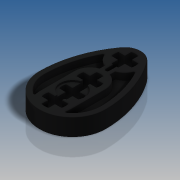
# Autodesk Inventor part: 6575-Black
Saved by Autodesk Inventor 2016 SP2 (Build 200236200, 236)
## iProperties
Created: 2015-01-12
Part Number: 6575-Black
Material: ABS Plastic
Document SubType Name: Modeling
Designer: D. Kohfeld
Density: 1.06 g/cm^3
Appearance: Black
Mass: 0.667179 g
Surface Area: 11.7051 cm^2
Volume: 0.629414 cm^3
Author: D. Kohfeld
Autodesk Inventor part; units mm, degrees
ref_plane "YZ Plane" through (0, 0, 0) normal (1, 0, 0) x (0, 1, 0)
ref_plane "XZ Plane" through (0, 0, 0) normal (0, 1, 0) x (-1, 0, 0)
ref_plane "XY Plane" through (0, 0, 0) normal (0, 0, 1) x (1, 0, 0)
sketch "Sketch2" plane through (0, 0, 0) normal (0, 1, 0) x (-1, 0, 0)
  arc A0 (7.5997, 3.9382) -> (-7.5997, 3.9382) centre (0, 4) ccw
  arc A1 (-2.894, -10.1412) -> (2.894, -10.1412) centre (0, -8) ccw
  arc A2 (2.894, -10.1412) -> (7.5997, 3.9382) centre (-16.3995, 4.1333) ccw
  arc A3 (-7.5997, 3.9382) -> (-2.894, -10.1412) centre (16.3995, 4.1333) ccw
  circle A4 centre (0, -8) radius 2.4 construction
  circle A5 centre (0, 8) radius 2.4 construction
  circle A6 centre (0, 4) radius 2.4 construction
  circle A7 centre (0, 0) radius 2.4 construction
  line L0 (-0.8, 10.2627) -> (-0.8, 8.8)
  line L1 (-0.8, 8.8) -> (-2.2627, 8.8)
  line L2 (-2.2627, 7.2) -> (-0.8, 7.2)
  line L3 (-0.8, 7.2) -> (-0.8, 4.8)
  line L4 (-0.8, 4.8) -> (-2.2627, 4.8)
  line L5 (-2.2627, 3.2) -> (-0.8, 3.2)
  line L6 (-0.8, 3.2) -> (-0.8, 0.8)
  line L7 (-0.8, 0.8) -> (-2.2627, 0.8)
  line L8 (-2.2627, -0.8) -> (-0.8, -0.8)
  line L9 (-0.8, -0.8) -> (-0.8, -2.2627)
  line L10 (0.8, -2.2627) -> (0.8, -0.8)
  line L11 (0.8, -0.8) -> (2.2627, -0.8)
  line L12 (2.2627, 0.8) -> (0.8, 0.8)
  line L13 (0.8, 0.8) -> (0.8, 3.2)
  line L14 (0.8, 3.2) -> (2.2627, 3.2)
  line L15 (2.2627, 4.8) -> (0.8, 4.8)
  line L16 (0.8, 4.8) -> (0.8, 7.2)
  line L17 (0.8, 7.2) -> (2.2627, 7.2)
  line L18 (2.2627, 8.8) -> (0.8, 8.8)
  line L19 (0.8, 8.8) -> (0.8, 10.2627)
  arc A8 (0.8, 10.2627) -> (-0.8, 10.2627) centre (0, 8) ccw
  arc A9 (-2.2627, 8.8) -> (-2.2627, 7.2) centre (0, 8) ccw
  arc A10 (2.2627, 7.2) -> (2.2627, 8.8) centre (0, 8) ccw
  arc A11 (2.2627, 3.2) -> (2.2627, 4.8) centre (0, 4) ccw
  arc A12 (-2.2627, 4.8) -> (-2.2627, 3.2) centre (0, 4) ccw
  arc A13 (-2.2627, 0.8) -> (-2.2627, -0.8) centre (0, 0) ccw
  arc A14 (-0.8, -2.2627) -> (0.8, -2.2627) centre (0, 0) ccw
  arc A15 (2.2627, -0.8) -> (2.2627, 0.8) centre (0, 0) ccw
  line L20 (-0.8, -5.7373) -> (-0.8, -7.2)
  line L21 (-0.8, -7.2) -> (-2.2627, -7.2)
  line L22 (-2.2627, -8.8) -> (-0.8, -8.8)
  line L23 (-0.8, -8.8) -> (-0.8, -10.2627)
  line L24 (0.8, -10.2627) -> (0.8, -8.8)
  line L25 (0.8, -8.8) -> (2.2627, -8.8)
  line L26 (2.2627, -7.2) -> (0.8, -7.2)
  line L27 (0.8, -7.2) -> (0.8, -5.7373)
  arc A16 (-2.2627, -7.2) -> (-2.2627, -8.8) centre (0, -8) ccw
  arc A17 (-0.8, -10.2627) -> (0.8, -10.2627) centre (0, -8) ccw
  arc A18 (2.2627, -8.8) -> (2.2627, -7.2) centre (0, -8) ccw
  arc A19 (6.3998, 3.948) -> (-6.3998, 3.948) centre (0, 4) ccw
  arc A20 (1.9293, -9.4275) -> (6.3998, 3.948) centre (-16.3995, 4.1333) ccw
  arc A21 (-1.9293, -9.4275) -> (1.9293, -9.4275) centre (0, -8) ccw
  arc A22 (-6.3998, 3.948) -> (-1.9293, -9.4275) centre (16.3995, 4.1333) ccw
  line L28 (-3.6, 8) -> (-3.6, 0)
  line L29 (3.6, 0) -> (3.6, 8)
  arc A23 (3.6, 8) -> (3.2726, 9.5) centre (0, 8) ccw
  arc A24 (-3.2726, 9.5) -> (-3.6, 8) centre (0, 8) ccw
  line L30 (-1.2, -4.6059) -> (-1.2, -3.3941)
  line L31 (1.2, -4.6059) -> (1.2, -3.3941)
  line L32 (-0.4, -5.6336) -> (-0.4, -4)
  arc A25 (0.4, -4) -> (-0.4, -4) centre (0, -4) ccw
  line L33 (0.4, -4) -> (0.4, -5.6336)
  arc A26 (0.8, -5.7373) -> (0.4, -5.6336) centre (0, -8) ccw
  arc A27 (-0.4, -5.6336) -> (-0.8, -5.7373) centre (0, -8) ccw
  arc A28 (-3.6, 0) -> (-1.2, -3.3941) centre (0, 0) ccw
  arc A29 (1.2, -3.3941) -> (3.6, 0) centre (0, 0) ccw
  arc A30 (3.4714, -7.0465) -> (1.2, -4.6059) centre (0, -8) ccw
  arc A31 (-1.2, -4.6059) -> (-3.4714, -7.0465) centre (0, -8) ccw
  dimension "d4" = 4.8
  dimension "d0" = 15.2
  dimension "d1" = 12
  dimension "d2" = 7.2
  dimension "d3" = 24
  dimension "d5" = 4
  dimension "d6" = 4
  dimension "d7" = 1.6
  dimension "d8" = 1.2
  dimension "d9" = 0.8
  dimension "d10" = 2.4
  dimension "d11" = 4
  constraints: 76 point on circle, 68 end point, 31 centre point, 25 equal length, 19 parallel, 12 perpendicular, 10 concentric, 10 tangent, 7 coincident, 7 vertical alignment, 5 equal radius, 3 vertical, 1 horizontal alignment, 19 other
  measures "d0" diameter of A0
  measures "d1" distance of A1.centre A0.centre
  measures "d2" diameter of A1
  measures "d3" radius of A3
  measures "d5" distance of A5.centre A0.centre
  measures "d6" distance of A7.centre A0.centre
  measures "d7" distance between parallel lines of L19 L0
  measures "d8" radial gap between concentric circles of A3 A22
  measures "d9" distance between parallel lines of L33 L32
  measures "d10" distance between parallel lines of L30 L31
  measures "d11" distance of A1.centre A25.centre
extrude "Extrusion1" add sketch "Sketch2" along normal mid plane 0.8 contours A19 A20 A30 L31 A29 L29 A23 | A24 L28 A28 L30 A31 A22 A19
extrude "Extrusion2" add sketch "Sketch2" along normal mid plane 4 contours A2 A1 A3 A0 | A19 A23 L29 A29 L31 A30 A20 A21 L24 L25 A18 L26 L27 A26 L33 A25 L32 A27 L20 L21 A16 L22 L23 A22 A31 L30 A28 L28 A24
sketch "Sketch3" plane through (0, 2, 0) normal (0, 1, 0) x (1, 0, 0)
  arc A0 (-7.5997, -3.9382) -> (7.5997, -3.9382) centre (0, -4) ccw projected
  circle A1 centre (0, -4) radius 2.8
  point P0 (0, 0)
  dimension "d17" = 5.6
  constraints: 1 centre point, 1 coincident
  measures "d17" diameter of A1
extrude "Extrusion3" cut sketch "Sketch3" against normal blind 0.4
fillet "Fillet1" radius 0.1 36 edges at (6.3628, 2, -3.4745) (0, 2, -11.6) (-6.3628, 2, -3.4745) (0, 2, 11.6) (0, -2, 11.6) (-6.3628, -2, -3.4745) (0, -2, -11.6) (6.3628, -2, -3.4745) (2.9394, 2, -2.0785) (3.5172, 2, 8.7677) (3.6, 2, 4) (-3.6, 2, 4) (-3.5172, 2, 8.7677) (-2.9394, 2, -2.0785) (-2.6353, 2, -5.5474) (1.2, 2, -4) (-1.2, 2, -4) (2.6353, 2, -5.5474) (5.5763, 2, 7.1408) (5.6324, 2, -1.7349) (-5.5763, 2, 7.1408) (-5.6324, 2, -1.7349) (5.6324, -2, -1.7349) (5.5763, -2, 7.1408) (3.5172, -2, 8.7677) (2.9394, -2, -2.0785) (3.6, -2, 4) (1.2, -2, -4) (2.6353, -2, -5.5474) (-2.6353, -2, -5.5474) (-1.2, -2, -4) (-3.6, -2, 4) (-3.5172, -2, 8.7677) (-2.9394, -2, -2.0785) (-5.6324, -2, -1.7349) (-5.5763, -2, 7.1408)
fillet "Fillet1" radius 0.2 8 edges at (-3.2726, 1.2, 9.5) (3.2726, 1.2, 9.5) (3.4714, 1.2, -7.0465) (-3.4714, 1.2, -7.0465) (3.4714, -1.2, -7.0465) (-3.4714, -1.2, -7.0465) (-3.2726, -1.2, 9.5) (3.2726, -1.2, 9.5)
equation "\"d4\" = tpd"
equation "\"d2\" = tlad"
equation "\"d5\" = 0.5 * lu"
equation "\"d6\" = d5"
equation "\"d7\" = axlet"
equation "\"d15\" = 0.5 * lu"
equation "\"d20\" = lf"
equation "\"tpd\" = 4.8"
equation "\"tlad\" = 7.2"
equation "\"lu\" = 8"
equation "\"axlet\" = 1.6"
equation "\"lf\" = 0.1"
body "Solid1"
